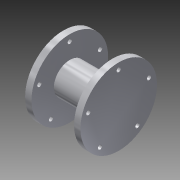
# Autodesk Inventor part: tool_1
Saved by Autodesk Inventor 2015 (Build 190159000, 159)
## iProperties
Created: 2015-12-22
Part Number: tool_1
Material: アルミニウム 6061
Document SubType Name: Modeling
Designer: Ryo
Density: 2.7 g/cm^3
Appearance: アルミニウム - フラット
Author: Ryo
Autodesk Inventor part; units mm, degrees
ref_plane "YZ Plane" through (0, 0, 0) normal (1, 0, 0) x (0, 1, 0)
ref_plane "XZ Plane" through (0, 0, 0) normal (0, 1, 0) x (-1, 0, 0)
ref_plane "XY Plane" through (0, 0, 0) normal (0, 0, 1) x (1, 0, 0)
sketch "スケッチ1" plane through (0, 0, 0) normal (1, 0, 0) x (0, 1, 0)
  circle A0 centre (0, 0) radius 36
  dimension "d0" = 72
  constraints: 1 centre point, 1 coincident
  measures "d0" diameter of A0
extrude "押し出し1" add sketch "スケッチ1" along normal blind 6
sketch "スケッチ2" plane through (6, 0, 0) normal (1, 0, 0) x (0, 0, -1)
  circle A0 centre (0, 0) radius 15
  dimension "d3" = 30
  constraints: 1 centre point, 1 coincident
  measures "d3" diameter of A0
extrude "押し出し2" add sketch "スケッチ2" along normal blind 40
sketch "スケッチ3" plane through (46, 0, 0) normal (1, 0, 0) x (0, 0, -1)
  circle A0 centre (0, 0) radius 36
  dimension "d6" = 72
  constraints: 1 centre point, 1 coincident
  measures "d6" diameter of A0
extrude "押し出し3" add sketch "スケッチ3" along normal blind 6
sketch "スケッチ4" plane through (0, 0, 0) normal (-1, 0, 0) x (0, 0, 1)
  circle A0 centre (30, 0) radius 2
  circle A1 centre (9.2705, 28.5317) radius 2
  circle A2 centre (-24.2705, 17.6336) radius 2
  circle A3 centre (-24.2705, -17.6336) radius 2
  circle A4 centre (9.2705, -28.5317) radius 2
  circle A5 centre (0, 0) radius 10
  dimension "d9" = 30
  dimension "d10" = 4
  dimension "d13" = 360
  dimension "d17" = 20
  constraints: 6 centre point, 1 coincident, 11 other
  measures "d9" distance of point (0, 0) A0.centre
  measures "d10" diameter of A0
  measures "d17" diameter of A5
extrude "押し出し4" cut sketch "スケッチ4" against normal blind 6 contours A0 | A1 | A2 | A3 | A4
extrude "押し出し5" add sketch "スケッチ4" along normal blind 2 contours A5
chamfer "面取り1" distance 1 angle 45 1 edges at (-2, 0, -10)
sketch "スケッチ6" plane through (52, 0, 0) normal (1, 0, 0) x (0, 0, -1)
  circle A0 centre (24.2705, 17.6336) radius 2 projected
  circle A1 centre (24.2705, 17.6336) radius 2 projected
  circle A2 centre (-9.2705, 28.5317) radius 2 projected
  circle A3 centre (-9.2705, 28.5317) radius 2 projected
  circle A4 centre (-30, 0) radius 2 projected
  circle A5 centre (24.2705, -17.6336) radius 2 projected
  circle A6 centre (24.2705, -17.6336) radius 2 projected
  circle A7 centre (-9.2705, -28.5317) radius 2 projected
  circle A8 centre (-9.2705, -28.5317) radius 2 projected
  point P0 (0, 0)
extrude "押し出し6" cut sketch "スケッチ6" against normal blind 6
